shell (Autodesk Fusion 360 design; units mm, degrees)
Autodesk Fusion 360 part; units mm, degrees
ref_plane "WorkPlane1" through (0, 0, 13.5) normal (0, 0, 1) x (1, 0, 0)
sketch "Sketch1" plane through (0, 0, 13.5) normal (0, 0, 1) x (1, 0, 0)
  circle A0 centre (0, 0) radius 9.5
  circle A1 centre (0, 0) radius 8.5
  line L0 (0, 0) -> (0, 20.5) construction
  circle A2 centre (0, 20.5) radius 6.1
  line L1 (0, 20.5) -> (0, 41) construction
  line L2 (12.5, -14.5) -> (-12.5, -14.5)
  line L3 (-12.5, -14.5) -> (-12.5, 55.5)
  line L4 (-12.5, 55.5) -> (12.5, 55.5)
  line L5 (12.5, 55.5) -> (12.5, -14.5)
  line L6 (12.5, -14.5) -> (-12.5, 55.5) construction
  line L7 (-12.5, -14.5) -> (12.5, 55.5) construction
  line L8 (4.25, 36.75) -> (-4.25, 36.75) construction
  line L9 (-4.25, 36.75) -> (-4.25, 45.25) construction
  line L10 (-4.25, 45.25) -> (4.25, 45.25) construction
  line L11 (4.25, 45.25) -> (4.25, 36.75) construction
  line L12 (4.25, 36.75) -> (-4.25, 45.25) construction
  line L13 (-4.25, 36.75) -> (4.25, 45.25) construction
  circle A3 centre (-4.25, 45.25) radius 1.25
  circle A4 centre (-4.25, 36.75) radius 1.25
  circle A5 centre (4.25, 36.75) radius 1.25
  circle A6 centre (4.25, 45.25) radius 1.25
  line L14 (12.5, 45.5) -> (32.5, 45.5)
  line L15 (32.5, 45.5) -> (32.5, 5.5)
  line L16 (32.5, 5.5) -> (12.5, 5.5)
  line L17 (12.5, 5.5) -> (12.5, 45.5)
  line L18 (-12.5, 45.5) -> (-32.5, 45.5)
  line L19 (-32.5, 45.5) -> (-32.5, 5.5)
  line L20 (-32.5, 5.5) -> (-12.5, 5.5)
  line L21 (-12.5, 5.5) -> (-12.5, 45.5)
  line L22 (12.5, -14.5) -> (32.5, -14.5)
  line L23 (32.5, -14.5) -> (32.5, -4.5)
  line L24 (32.5, -4.5) -> (12.5, -4.5)
  line L25 (12.5, -4.5) -> (12.5, -14.5)
  line L26 (-12.5, -14.5) -> (-32.5, -14.5)
  line L27 (-32.5, -14.5) -> (-32.5, -4.5)
  line L28 (-32.5, -4.5) -> (-12.5, -4.5)
  line L29 (-12.5, -4.5) -> (-12.5, -14.5)
  point P0 (0, 20.5)
  point P1 (0, 41)
  dimension "d2" = 1
  dimension "d3" = 20.5
  dimension "d4" = 12.2
  dimension "d5" = 20.5
  dimension "d6" = 25
  dimension "d7" = 70
  dimension "d10" = 8.5
  dimension "d11" = 8.5
  dimension "d12" = 2.5
  dimension "d14" = 360
  dimension "d68" = 10
  dimension "d69" = 20
  dimension "d70" = 20
  dimension "d71" = 10
  constraint concentric A0 A1
  constraint coincident A0.centre A1.centre
  constraint vertical L0
  constraint coincident P0 L0.end
  constraint parallel L0 L1
  constraint horizontal L2
  constraint perpendicular L2 L3
  constraint parallel L2 L4
  constraint parallel L3 L5
  constraint coincident L6 P0
  constraint coincident L7 P0
  constraint horizontal L8
  constraint perpendicular L8 L9
  constraint parallel L8 L10
  constraint parallel L9 L11
  constraint coincident L12 P1
  constraint coincident L13 P1
  constraint coincident P1 L1.end
  constraint coincident L9.end L10.start
  constraint horizontal L14
  constraint vertical L15
  constraint horizontal L16
  constraint vertical L17
  constraint coincident L5 L14.start
  constraint horizontal L18
  constraint vertical L19
  constraint horizontal L20
  constraint vertical L21
  constraint coincident L3 L18.start
  constraint collinear L14 L18
  constraint collinear L16 L20
  constraint equal L16 L20
  constraint horizontal L22
  constraint vertical L23
  constraint horizontal L24
  constraint vertical L25
  constraint horizontal L26
  constraint vertical L27
  constraint horizontal L28
  constraint vertical L29
  constraint collinear L15 L23
  constraint collinear L19 L27
  constraint collinear L24 L28
  measures "d2" distance of A0 A1
  measures "d3" distance of A0.centre P0
  measures "d4" diameter of A2
  measures "d5" distance of P0 P1
  measures "d6" distance of L3.end L4.end
  measures "d7" distance of L2.end L3.end
  measures "d10" distance of L9.end L10.end
  measures "d11" distance of L8.end L9.end
  measures "d12" diameter of A3
  measures "d68" distance of L4.end L14
  measures "d69" distance of L2.start L16
  measures "d70" distance of L15.end L16.end
  measures "d71" distance of L22.end L23.end
extrude "Extrude1" add sketch "Sketch1" along normal blind 4 contours L2 L3 L4 L5 L17 L21 L25 L29
sketch "Sketch2" plane through (0, 55.5, 0) normal (0, 1, 0) x (-1, 0, 0)
  line L0 (-12.5, 13.5) -> (12.5, 13.5)
  line L1 (12.5, 13.5) -> (12.5, 17.5)
  line L2 (12.5, 17.5) -> (-12.5, 17.5)
  line L3 (-12.5, 17.5) -> (-12.5, 13.5)
  circle A0 centre (25, 6.75) radius 3
  circle A1 centre (-25, 6.75) radius 3
  circle A2 centre (25, 6.75) radius 5
  circle A3 centre (-25, 6.75) radius 5
  line L4 (28.5355, 10.2855) -> (21.3211, 17.5)
  line L5 (21.3211, 17.5) -> (12.5, 17.5)
  line L6 (-12.5, 17.5) -> (-21.3211, 17.5)
  line L7 (-21.3211, 17.5) -> (-28.5355, 10.2855)
  line L8 (28.5355, 10.2855) -> (25, 6.75) construction
  line L9 (-25, 6.75) -> (-28.5355, 10.2855) construction
  line L10 (12.5, 13.5) -> (20, 13.5)
  line L11 (20, 13.5) -> (20, 6.75)
  line L12 (-12.5, 13.5) -> (-20, 13.5)
  line L13 (-20, 13.5) -> (-20, 6.75)
  dimension "d62" = 2
  dimension "d63" = 2
  dimension "d64" = 135
  dimension "d65" = 135
  constraint coincident A2 L4.start
  constraint coincident L1.end L2.start
  constraint coincident L2.end L3.start
  constraint perpendicular L3 L6
  constraint coincident A3 L7.end
  constraint tangent A3 L7
  constraint collinear L2 L5
  constraint coincident A0.centre A2.centre
  constraint perpendicular L4 L8
  constraint coincident A1.centre A3.centre
  constraint coincident L0.end L1.start
  constraint perpendicular L1 L10
  constraint coincident A2 L11.end
  constraint tangent A2 L11
  constraint coincident L0.start L3.end
  constraint perpendicular L3 L12
  constraint coincident A3 L13.end
  constraint tangent A3 L13
  constraint perpendicular L10 L11
  constraint perpendicular L12 L13
  measures "d64" angle of L4 L5
  measures "d65" angle of L6 L7
extrude "Extrude2" add sketch "Sketch2" against normal up to surface (70 mm away) contours L3 A3 L6 L7 L12 L13 | L1 A2 L4 L5 L10 L11 | A3 | A2
extrude "Extrude3" cut sketch "Sketch1" along normal blind 5 and the other way blind 15 contours L5 L22 L23 L24 L25 | L3 L26 L27 L28 L29 | L5 L14 L15 L16 L17 | L3 L18 L19 L20 L21
fillet "Fillet1" radius 5 4 edges at (20, 50.5, 13.5) (20, 0.5, 13.5) (-20, 50.5, 13.5) (-20, 0.5, 13.5)
sketch "Sketch3" plane through (0, 0, 17.5) normal (0, 0, 1) x (-1, 0, 0)
  line L0 (-12.5, -45.5) -> (-21.3211, -45.5)
  line L1 (-21.3211, -45.5) -> (-21.3211, -55.5)
  line L2 (-21.3211, -55.5) -> (21.3211, -55.5)
  line L3 (21.3211, -55.5) -> (21.3211, -45.5)
  line L4 (21.3211, -45.5) -> (12.5, -45.5)
  line L5 (12.5, -45.5) -> (12.5, -5.5)
  line L6 (12.5, -5.5) -> (21.3211, -5.5)
  line L7 (21.3211, -5.5) -> (21.3211, 4.5)
  line L8 (21.3211, 4.5) -> (12.5, 4.5)
  line L9 (12.5, 4.5) -> (12.5, 14.5)
  line L10 (12.5, 14.5) -> (-12.5, 14.5)
  line L11 (-12.5, 14.5) -> (-12.5, 4.5)
  line L12 (-12.5, 4.5) -> (-21.3211, 4.5)
  line L13 (-21.3211, 4.5) -> (-21.3211, -5.5)
  line L14 (-21.3211, -5.5) -> (-12.5, -5.5)
  line L15 (-12.5, -5.5) -> (-12.5, -45.5)
  circle A0 centre (4.25, -45.25) radius 1.25
  circle A1 centre (0, -20.5) radius 6.1
  circle A2 centre (4.25, -36.75) radius 1.25
  circle A3 centre (-4.25, -36.75) radius 1.25
  circle A4 centre (-4.25, -45.25) radius 1.25
  circle A5 centre (0, 0) radius 9.5
  circle A6 centre (4.25, -45.25) radius 2
  circle A7 centre (-4.25, -45.25) radius 2
  circle A8 centre (4.25, -36.75) radius 2
  circle A9 centre (-4.25, -36.75) radius 2
  dimension "d83" = 4
  dimension "d84" = 4
  dimension "d85" = 4
  dimension "d86" = 4
  constraint concentric A0 A6
  constraint concentric A4 A7
  constraint concentric A2 A8
  constraint concentric A3 A9
  measures "d83" diameter of A6
  measures "d84" diameter of A7
  measures "d85" diameter of A8
  measures "d86" diameter of A9
extrude "Extrude4" cut sketch "Sketch3" against normal blind 0.5 contours A6 | A7 | A8 | A9
extrude "Extrude5" cut 2 faces at (-16.5109, 45.5, 16.1497) (16.5109, 45.5, 16.1497) along direction (0, 1, 0) blind 0.1
sketch "Sketch4" plane through (0, 0, 13.5) normal (0, 0, -1) x (1, 0, 0)
  circle A0 centre (0, 0) radius 9.5
  circle A1 centre (4.25, -45.25) radius 1.25
  circle A2 centre (4.25, -36.75) radius 1.25
  circle A3 centre (-4.25, -45.25) radius 1.25
  circle A4 centre (-4.25, -36.75) radius 1.25
  circle A5 centre (0, -20.5) radius 6.1
  line L0 (-12.5, -5.5) -> (-12.5, -45.6)
  line L1 (-12.5, -45.6) -> (-15, -45.6)
  line L2 (-15, -45.6) -> (-15, -55.5)
  line L3 (-15, -55.5) -> (15, -55.5)
  line L4 (15, -55.5) -> (15, -45.6)
  line L5 (15, -45.6) -> (12.5, -45.6)
  line L6 (12.5, -45.6) -> (12.5, -5.5)
  line L7 (12.5, -5.5) -> (15, -5.5)
  line L8 (15, -5.5) -> (15, 4.5)
  line L9 (15, 4.5) -> (12.5, 4.5)
  line L10 (12.5, 4.5) -> (12.5, 14.5)
  line L11 (12.5, 14.5) -> (-12.5, 14.5)
  line L12 (-12.5, 14.5) -> (-12.5, 4.5)
  line L13 (-12.5, 4.5) -> (-15, 4.5)
  line L14 (-15, 4.5) -> (-15, -5.5)
  line L15 (-15, -5.5) -> (-12.5, -5.5)
  circle A6 centre (0, 0) radius 15
  dimension "d207" = 30
  constraint coincident A0.centre A6.centre
  measures "d207" diameter of A6
extrude "Extrude6" cut sketch "Sketch4" against normal blind 0.5 contours A5 L0 L6 L7 L9 L10 L11 L12 L13 L15 A6 | L11 A6
sketch "Sketch5" plane through (0, 0, 17.5) normal (0, 0, 1) x (-1, 0, 0)
  circle A0 centre (0, 0) radius 9.5
  circle A1 centre (0, -20.5) radius 6.1
  circle A2 centre (-4.25, -45.25) radius 2
  circle A3 centre (4.25, -45.25) radius 2
  circle A4 centre (4.25, -36.75) radius 2
  circle A5 centre (-4.25, -36.75) radius 2
  line L0 (21.3211, -45.6) -> (12.5, -45.6)
  line L1 (12.5, -45.6) -> (12.5, -5.5)
  line L2 (12.5, -5.5) -> (21.3211, -5.5)
  line L3 (21.3211, -5.5) -> (21.3211, 4.5)
  line L4 (21.3211, 4.5) -> (12.5, 4.5)
  line L5 (12.5, 4.5) -> (12.5, 14.5)
  line L6 (12.5, 14.5) -> (-12.5, 14.5)
  line L7 (-12.5, 14.5) -> (-12.5, 4.5)
  line L8 (-12.5, 4.5) -> (-21.3211, 4.5)
  line L9 (-21.3211, 4.5) -> (-21.3211, -5.5)
  line L10 (-21.3211, -5.5) -> (-12.5, -5.5)
  line L11 (-12.5, -5.5) -> (-12.5, -45.6)
  line L12 (-12.5, -45.6) -> (-21.3211, -45.6)
  line L13 (-21.3211, -45.6) -> (-21.3211, -55.5)
  line L14 (-21.3211, -55.5) -> (21.3211, -55.5)
  line L15 (21.3211, -55.5) -> (21.3211, -45.6)
  line L16 (-9.5, 0) -> (-9.5, 4.5)
  line L17 (-9.5, 4.5) -> (-12.5, 4.5)
  line L18 (9.5, 0) -> (9.5, 4.5)
  line L19 (9.5, 4.5) -> (12.5, 4.5)
  constraint coincident A0 L16.start
  constraint tangent A0 L16
  constraint perpendicular L6 L16
  constraint coincident L7.end L8.start
  constraint coincident A0 L18.start
  constraint tangent A0 L18
  constraint parallel L16 L18
  constraint coincident L4.end L5.start
  constraint perpendicular L5 L19
  constraint perpendicular L16 L17
extrude "Extrude7" cut sketch "Sketch5" against normal blind 5 contours A0 L5 L6 L7 L16 L17 L18 L19
